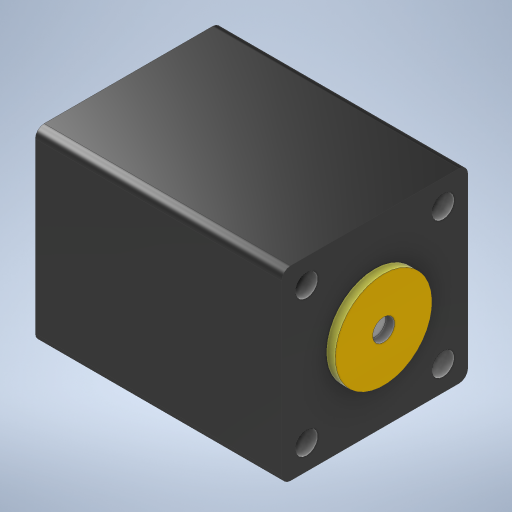
# Autodesk Inventor part: stepper
Saved by Autodesk Inventor 2023.2 (Build 272271030, 271C)
## iProperties
Created: 2023-03-04
Part Number: stepper
Material: Generic
Document SubType Name: Modeling
Designer: Cris Pat
Density: 1 g/cm^3
Appearance: Default
Author: Cris Pat
Autodesk Inventor part; units mm, degrees
ref_plane "XZ Plane" through (0, 0, 0) normal (0, 1, 0) x (-1, 0, 0)
ref_plane "XY Plane" through (0, 0, 0) normal (0, 0, 1) x (1, 0, 0)
sketch "Sketch1" plane through (0, 0, 0) normal (1, 0, 0) x (0, 1, 0)
  line L0 (-21.15, 21.15) -> (21.15, 21.15)
  line L1 (21.15, 21.15) -> (21.15, -21.15)
  line L2 (21.15, -21.15) -> (-21.15, -21.15)
  line L3 (-21.15, -21.15) -> (-21.15, 21.15)
  point P0 (0, 0)
  point P1 (0, 21.15)
  point P2 (21.15, 0)
  dimension "d0" = 42.3
  dimension "d1" = 42.3
  constraints: 8 end point, 2 midpoint, 2 parallel, 1 horizontal, 1 horizontal alignment, 1 perpendicular, 1 vertical alignment
  measures "d0" distance of L1.end L2.end
  measures "d1" distance of L0.end L1.end
extrude "Extrusion1" add sketch "Sketch1" along normal mid plane 56
ref_plane "Work Plane1" through (28, 0, 0) normal (1, 0, 0) x (0, 1, 0)
sketch "Sketch2" plane through (28, 0, 0) normal (1, 0, 0) x (0, 1, 0)
  circle A0 centre (0, 0) radius 11
  circle A1 centre (0, 0) radius 2.5
  circle A2 centre (15.5, 15.5) radius 2.55
  line L0 (21.15, -21.15) -> (21.15, 21.15) construction
  line L1 (21.15, 0) -> (0, 0) construction
  line L2 (0, 0) -> (0, 21.15) construction
  line L3 (21.15, 21.15) -> (-21.15, 21.15) construction
  circle A3 centre (15.5, -15.5) radius 2.55
  circle A4 centre (-15.5, 15.5) radius 2.55
  circle A5 centre (-15.5, -15.5) radius 2.55
  line L4 (1, 2.2913) -> (1, -2.2913)
  dimension "d5" = 22
  dimension "d6" = 5
  dimension "d15" = 5.1
  dimension "d16" = 31
  dimension "d17" = 31
  dimension "d20" = 1
  constraints: 6 centre point, 6 end point, 3 symmetric about line, 2 coincident, 2 midpoint, 2 point on circle, 1 perpendicular, 1 vertical, 3 other
  measures "d5" diameter of A0
  measures "d6" diameter of A1
  measures "d15" diameter of A2
  measures "d16" distance of A3.centre A2.centre
  measures "d17" distance of A4.centre A2.centre
  measures "d20" distance from line of L4 point (0, 0)
extrude "Extrusion2" add sketch "Sketch2" along normal blind 2 contours A0
fillet "Fillet1" radius 2 1 edges at (0, 21.15, 21.15)
pattern_circular "Circular Pattern1" count 4 over 360 about axis through (28, 0, 0) along (1, 0, 0) of "Fillet1"
extrude "Extrusion4" cut sketch "Sketch2" against normal through all contours A2 | A3 | A4 | A5
body "Solid1"
